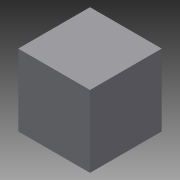
# Autodesk Inventor part: 测试零件1
Saved by Autodesk Inventor 2014 (Build 180170000, 170)
## iProperties
Created: 2016-04-03
Part Number: 测试零件1
Material: 常规
Document SubType Name: Modeling
Designer: HouZhimin
Density: 1 g/cm^3
Appearance: 默认
Author: HouZhimin
Autodesk Inventor part; units mm, degrees
ref_plane "YZ Plane" through (0, 0, 0) normal (1, 0, 0) x (0, 1, 0)
ref_plane "XZ Plane" through (0, 0, 0) normal (0, 1, 0) x (-1, 0, 0)
ref_plane "XY Plane" through (0, 0, 0) normal (0, 0, 1) x (1, 0, 0)
sketch "草图1" plane through (0, 0, 0) normal (0, 0, 1) x (1, 0, 0)
  line L0 (0, 0) -> (200, 0)
  line L1 (200, 0) -> (200, 200)
  line L2 (200, 200) -> (0, 200)
  line L3 (0, 200) -> (0, 0)
  constraints: 8 end point, 2 parallel, 1 horizontal, 1 perpendicular
extrude "拉伸1" add sketch "草图1" along normal blind 200
